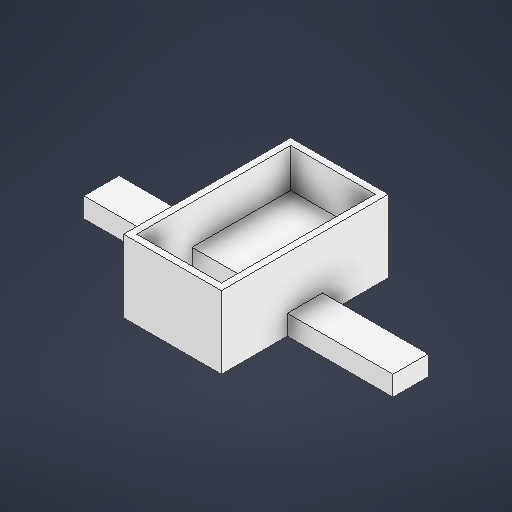
# Autodesk Inventor part: HorizontalRotationServoHolder
Saved by Autodesk Inventor 2025 (Build 290162000, 162)
## iProperties
Created: 2024-04-23
Part Number: HorizontalRotationServoHolder
Material: Generic
Document SubType Name: Modeling
Designer: conno
Density: 1 g/cm^3
Appearance: Default
Author: conno
Autodesk Inventor part; units mm, degrees
ref_plane "YZ Plane" through (0, 0, 0) normal (1, 0, 0) x (0, 1, 0)
ref_plane "XZ Plane" through (0, 0, 0) normal (0, 1, 0) x (-1, 0, 0)
ref_plane "XY Plane" through (0, 0, 0) normal (0, 0, 1) x (1, 0, 0)
sketch "Sketch1" plane through (0, 0, 0) normal (0, 1, 0) x (-1, 0, 0)
  line L0 (9.779, 18.10385) -> (-9.779, 18.10385)
  line L1 (-9.779, 18.10385) -> (-9.779, -18.10385)
  line L2 (-9.779, -18.10385) -> (9.779, -18.10385)
  line L3 (9.779, -18.10385) -> (9.779, 18.10385)
  line L4 (9.779, 18.10385) -> (-9.779, -18.10385) construction
  line L5 (-9.779, 18.10385) -> (9.779, -18.10385) construction
  point P0 (0, 0)
  dimension "d0" = 19.558
  dimension "d1" = 36.2077
  constraints: 12 end point, 2 midpoint, 2 parallel, 1 horizontal, 1 perpendicular
  measures "d0" distance of L2.end L1.end
  measures "d1" distance of L1.end L0.end
extrude "Base" add sketch "Sketch1" along normal blind 1.5875
sketch "Sketch2" plane through (0, 1.5875, 0) normal (0, 1, 0) x (1, 0, 0)
  line L0 (-9.779, 18.10385) -> (-9.779, -18.10385)
  line L1 (-9.779, -10.16635) -> (9.779, -10.16635)
  line L2 (9.779, -18.10385) -> (9.779, 18.10385)
  line L3 (-9.779, -18.10385) -> (9.779, -18.10385)
  line L4 (-9.779, -5.40385) -> (9.779, -5.40385)
  line L5 (9.779, 18.10385) -> (-9.779, 18.10385)
  point P0 (0, 0)
  dimension "d4" = 7.9375
  dimension "d5" = 4.7625
  constraints: 4 end point, 4 point on line, 1 horizontal, 1 perpendicular
  measures "d4" distance between parallel lines of L3 L1
  measures "d5" distance between parallel lines of L4 L1
extrude "Tab Indent" add sketch "Sketch2" along normal blind 6.4389 contours L5 L2 L4 L0 | L1 L2 L3 L0
thicken "Outward Servo Body Offset" operation add thickness 0.396875 both sides no extend neighbours no toward (0, 0, 1) faces at (-3.259667, 5.350933, 18.10385) (9.779, 3.204633, -10.26795) (-9.779, 3.204633, -10.26795) (3.259667, 5.350933, -18.10385)
thicken "Inwawrd Servo Tab Offset" operation cut thickness 0.198437 both sides no extend neighbours no toward (0, -1, 0) faces at (3.391958, 1.5875, 8.57885) (3.391958, 5.8801, 10.16635) (-3.391958, 3.7338, 5.40385)
sketch "Sketch3" plane through (0, 0, 0) normal (0, -1, 0) x (1, 0, 0)
  line L0 (10.175875, -18.500725) -> (-10.175875, -18.500725)
  line L1 (-10.175875, -18.500725) -> (-10.175875, 5.205413)
  line L2 (-10.175875, 10.364787) -> (-10.175875, 5.205413)
  line L3 (-10.175875, 10.364787) -> (-10.175875, 18.500725)
  line L4 (-10.175875, 18.500725) -> (10.175875, 18.500725)
  line L5 (10.175875, 18.500725) -> (10.175875, 10.364787)
  line L6 (10.175875, 5.205412) -> (10.175875, 10.364787)
  line L7 (10.175875, 5.205412) -> (10.175875, -18.500725)
  line L8 (-11.763375, -20.088225) -> (11.763375, -20.088225)
  line L9 (11.763375, -20.088225) -> (11.763375, 5.8166)
  line L10 (11.763375, 5.8166) -> (11.763375, 9.9187)
  line L11 (11.763375, 9.9187) -> (11.763375, 20.088225)
  line L12 (11.763375, 20.088225) -> (-11.763375, 20.088225)
  line L13 (-11.763375, 20.088225) -> (-11.763375, 10.315575)
  line L14 (-11.763375, 10.315575) -> (-11.763375, 6.213475)
  line L15 (-11.763375, 6.213475) -> (-11.763375, -20.088225)
  point P0 (0, 0)
  dimension "d12" = 1.5875
  constraints: 16 end point, 7 other
  measures "d12" distance between parallel lines of L0 L8
extrude "Walls" add sketch "Sketch3" against normal blind 17.399
sketch "Sketch4" plane through (0, 0, 0) normal (0, -1, 0) x (1, 0, 0)
  line L0 (11.763375, -20.088225) -> (11.763375, 20.088225)
  line L1 (11.763375, 20.088225) -> (-11.763375, 20.088225)
  line L2 (-11.763375, 20.088225) -> (-11.763375, -20.088225)
  line L3 (-11.763375, -20.088225) -> (11.763375, -20.088225)
  line L4 (11.763375, 0) -> (-11.763375, 0) construction
  line L5 (11.763375, -4.233333) -> (37.163375, -4.233333)
  line L6 (37.163375, -4.233333) -> (37.163375, 4.233333)
  line L7 (37.163375, 4.233333) -> (11.763375, 4.233333)
  line L8 (11.763375, 4.233333) -> (11.763375, -4.233333)
  line L9 (-11.763375, -4.233333) -> (-37.163375, -4.233333)
  line L10 (-37.163375, -4.233333) -> (-37.163375, 4.233333)
  line L11 (-37.163375, 4.233333) -> (-11.763375, 4.233333)
  line L12 (-11.763375, 4.233333) -> (-11.763375, -4.233333)
  point P0 (0, 0)
  point P1 (11.763375, 4.233333)
  point P2 (-11.763375, 4.233333)
  dimension "d15" = 8.46667
  dimension "d16" = 8.46667
  dimension "d17" = 25.4
  dimension "d18" = 25.4
  constraints: 18 end point, 4 parallel, 2 horizontal, 2 midpoint, 2 perpendicular, 2 point on line, 2 other
  measures "d15" distance between parallel lines of L7 L5
  measures "d16" distance between parallel lines of L11 L9
  measures "d17" distance between parallel lines of L0 L6
  measures "d18" distance between parallel lines of L2 L10
extrude "Stabilization Legs" add sketch "Sketch4" against normal blind 4.7625 contours L0 L7 L6 L5 | L9 L10 L11 L2
equation "\"d0\" = ServoWidth"
equation "\"d1\" = ServoLength"
equation "\"d4\" = ServoTabDepthOffset"
equation "\"d5\" = ServoTabWidth"
equation "\"d6\" = ServoTabHeight"
equation "\"d16\" = d15"
equation "\"d17\" = d18"
equation "\"ServoWidth\" = 19.558"
equation "\"ServoLength\" = 36.2077"
equation "\"ServoTabDepthOffset\" = 7.9375"
equation "\"ServoTabWidth\" = 4.7625"
equation "\"ServoTabHeight\" = 6.4389"
body "Solid1"
